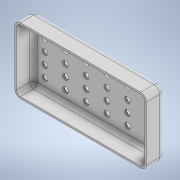
# Autodesk Inventor part: Peça2-Rubia
Saved by Autodesk Inventor 2021 (Build 250183000, 183)
## iProperties
Created: 2021-03-18
Part Number: Peça2-Rubia
Material: Genérico
Document SubType Name: Modeling
Designer: rubia
Density: 1 g/cm^3
Appearance: Padrão
Author: rubia
Autodesk Inventor part; units mm, degrees
ref_plane "YZ Plane" through (0, 0, 0) normal (1, 0, 0) x (0, 1, 0)
ref_plane "XZ Plane" through (0, 0, 0) normal (0, 1, 0) x (-1, 0, 0)
ref_plane "XY Plane" through (0, 0, 0) normal (0, 0, 1) x (1, 0, 0)
sketch "Esboço1" plane through (0, 0, 0) normal (0, 0, 1) x (1, 0, 0)
  line L0 (0, 0) -> (70, 0)
  line L1 (70, 0) -> (70, 35)
  line L2 (70, 35) -> (0, 35)
  line L3 (0, 35) -> (0, 0)
  dimension "d0" = 70
  dimension "d1" = 35
  constraints: 8 end point, 2 parallel, 1 horizontal, 1 perpendicular
  measures "d0" distance of L2.end L1.end
  measures "d1" distance of L1.end L0.end
extrude "Extrusão1" add sketch "Esboço1" along normal blind 10
fillet "Arredondamento1" radius 3 4 edges at (70, 35, 5) (70, 0, 5) (0, 35, 5) (0, 0, 5)
fillet "Arredondamento2" radius 3 8 edges at (0.8787, 34.1213, 0) (0, 17.5, 0) (0.8787, 0.8787, 0) (35, 0, 0) (69.1213, 0.8787, 0) (70, 17.5, 0) (69.1213, 34.1213, 0) (35, 35, 0)
shell "Casca1" thickness 1 removed faces 1 at (45.6667, 11.6667, 10)
sketch "Esboço2" plane through (0, 0, 0) normal (0, 0, -1) x (-1, 0, 0)
  circle A0 centre (-7, 7) radius 1.5
  line L0 (-3, 3) -> (-67, 3) projected
  line L1 (-3, 32) -> (-3, 3) projected
  point P0 (0, 0)
  dimension "d7" = 3
  dimension "d8" = 4
  dimension "d9" = 4
  constraints: 1 centre point
  measures "d7" diameter of A0
  measures "d8" distance from line of L0 A0.centre
  measures "d9" distance from line of L1 A0.centre
extrude "Extrusão2" cut sketch "Esboço2" against normal through all
pattern_linear "Padrão retangular1" count 6 spacing 11 along (1, 0, 0) count 4 spacing 6 along (0, 1, 0) of "Extrusão2"
